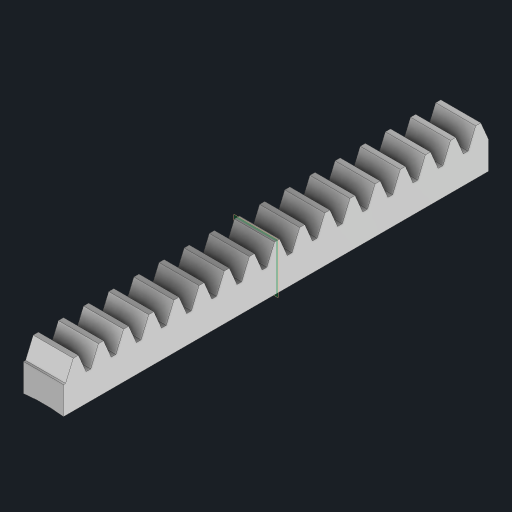
# Autodesk Inventor part: TAPA PRICIPAL CON CREMALLERA
Saved by Autodesk Inventor 2024.3 (Build 283343000, 343)
## iProperties
Created: 2024-06-13
Part Number: TAPA PRICIPAL CON CREMALLERA
Material: Generic
Document SubType Name: Modeling
Designer: Jhuliams
Density: 1 g/cm^3
Appearance: Default
Author: Jhuliams
Autodesk Inventor part; units mm, degrees
ref_plane "YZ Plane" through (0, 0, 0) normal (1, 0, 0) x (0, 1, 0)
ref_plane "XZ Plane" through (0, 0, 0) normal (0, 1, 0) x (-1, 0, 0)
ref_plane "XY Plane" through (0, 0, 0) normal (0, 0, 1) x (1, 0, 0)
sketch "Sketch4" plane through (0, 0, 0) normal (1, 0, 0) x (0, 1, 0)
  line L0 (0, -16.645) -> (0, -21.1217)
  line L1 (3, -17.923) -> (3, -19.8438)
  line L2 (3, -19.8438) -> (-3.75, -22.7192)
  line L3 (0, -21.1217) -> (0, -16.645)
  line L4 (0, -18.8834) -> (0.5045, -18.8834)
  line L5 (3, -17.923) -> (-3.75, -15.0476)
  line L6 (-3.75, 277.1181) -> (-10.75, 277.1181)
  line L7 (-10.75, 277.1181) -> (-10.75, -22.7192)
  line L8 (-10.75, -22.7192) -> (-3.75, -22.7192)
  line L9 (-3.75, -22.7192) -> (-3.75, 277.1181)
  line L10 (0, -7.2203) -> (0, -11.697)
  line L11 (3, -8.4983) -> (3, -10.419)
  line L12 (3, -10.419) -> (-3.75, -13.2945)
  line L13 (0, -11.697) -> (0, -7.2203)
  line L14 (0, -9.4587) -> (0.5045, -9.4587)
  line L15 (3, -8.4983) -> (-3.75, -5.6229)
  line L16 (0, 2.2044) -> (0, -2.2723)
  line L17 (3, 0.9264) -> (3, -0.9943)
  line L18 (3, -0.9943) -> (-3.75, -3.8698)
  line L19 (0, -2.2723) -> (0, 2.2044)
  line L20 (0, -0.034) -> (0.5045, -0.034)
  line L21 (3, 0.9264) -> (-3.75, 3.8018)
  line L22 (0, 11.6291) -> (0, 7.1524)
  line L23 (3, 10.3511) -> (3, 8.4304)
  line L24 (3, 8.4304) -> (-3.75, 5.5549)
  line L25 (0, 7.1524) -> (0, 11.6291)
  line L26 (0, 9.3907) -> (0.5045, 9.3907)
  line L27 (3, 10.3511) -> (-3.75, 13.2265)
  line L28 (0, 21.0538) -> (0, 16.5771)
  line L29 (3, 19.7758) -> (3, 17.8551)
  line L30 (3, 17.8551) -> (-3.75, 14.9796)
  line L31 (0, 16.5771) -> (0, 21.0538)
  line L32 (0, 18.8154) -> (0.5045, 18.8154)
  line L33 (3, 19.7758) -> (-3.75, 22.6512)
  line L34 (0, 30.4785) -> (0, 26.0018)
  line L35 (3, 29.2005) -> (3, 27.2797)
  line L36 (3, 27.2797) -> (-3.75, 24.4043)
  line L37 (0, 26.0018) -> (0, 30.4785)
  line L38 (0, 28.2401) -> (0.5045, 28.2401)
  line L39 (3, 29.2005) -> (-3.75, 32.0759)
  line L40 (0, 39.9032) -> (0, 35.4265)
  line L41 (3, 38.6252) -> (3, 36.7045)
  line L42 (3, 36.7045) -> (-3.75, 33.829)
  line L43 (0, 35.4265) -> (0, 39.9032)
  line L44 (0, 37.6648) -> (0.5045, 37.6648)
  line L45 (3, 38.6252) -> (-3.75, 41.5006)
  line L46 (0, 49.3279) -> (0, 44.8512)
  line L47 (3, 48.0499) -> (3, 46.1292)
  line L48 (3, 46.1292) -> (-3.75, 43.2537)
  line L49 (0, 44.8512) -> (0, 49.3279)
  line L50 (0, 47.0895) -> (0.5045, 47.0895)
  line L51 (3, 48.0499) -> (-3.75, 50.9253)
  line L52 (0, 58.7526) -> (0, 54.2759)
  line L53 (3, 57.4746) -> (3, 55.5539)
  line L54 (3, 55.5539) -> (-3.75, 52.6784)
  line L55 (0, 54.2759) -> (0, 58.7526)
  line L56 (0, 56.5142) -> (0.5045, 56.5142)
  line L57 (3, 57.4746) -> (-3.75, 60.35)
  line L58 (0, 68.1773) -> (0, 63.7006)
  line L59 (3, 66.8993) -> (3, 64.9785)
  line L60 (3, 64.9785) -> (-3.75, 62.1031)
  line L61 (0, 63.7006) -> (0, 68.1773)
  line L62 (0, 65.9389) -> (0.5045, 65.9389)
  line L63 (3, 66.8993) -> (-3.75, 69.7747)
  line L64 (0, 77.602) -> (0, 73.1253)
  line L65 (3, 76.324) -> (3, 74.4032)
  line L66 (3, 74.4032) -> (-3.75, 71.5278)
  line L67 (0, 73.1253) -> (0, 77.602)
  line L68 (0, 75.3636) -> (0.5045, 75.3636)
  line L69 (3, 76.324) -> (-3.75, 79.1994)
  line L70 (0, 87.0267) -> (0, 82.55)
  line L71 (3, 85.7487) -> (3, 83.828)
  line L72 (3, 83.828) -> (-3.75, 80.9525)
  line L73 (0, 82.55) -> (0, 87.0267)
  line L74 (0, 84.7883) -> (0.5045, 84.7883)
  line L75 (3, 85.7487) -> (-3.75, 88.6241)
  line L76 (0, 96.4514) -> (0, 91.9747)
  line L77 (3, 95.1734) -> (3, 93.2527)
  line L78 (3, 93.2527) -> (-3.75, 90.3772)
  line L79 (0, 91.9747) -> (0, 96.4514)
  line L80 (0, 94.213) -> (0.5045, 94.213)
  line L81 (3, 95.1734) -> (-3.75, 98.0488)
  line L82 (0, 105.8761) -> (0, 101.3994)
  line L83 (3, 104.5981) -> (3, 102.6774)
  line L84 (3, 102.6774) -> (-3.75, 99.8019)
  line L85 (0, 101.3994) -> (0, 105.8761)
  line L86 (0, 103.6377) -> (0.5045, 103.6377)
  line L87 (3, 104.5981) -> (-3.75, 107.4735)
  line L88 (0, 115.3008) -> (0, 110.8241)
  line L89 (3, 114.0228) -> (3, 112.1021)
  line L90 (3, 112.1021) -> (-3.75, 109.2266)
  line L91 (0, 110.8241) -> (0, 115.3008)
  line L92 (0, 113.0624) -> (0.5045, 113.0624)
  line L93 (3, 114.0228) -> (-3.75, 116.8982)
  line L94 (0, 124.7255) -> (0, 120.2488)
  line L95 (3, 123.4475) -> (3, 121.5268)
  line L96 (3, 121.5268) -> (-3.75, 118.6513)
  line L97 (0, 120.2488) -> (0, 124.7255)
  line L98 (0, 122.4871) -> (0.5045, 122.4871)
  line L99 (3, 123.4475) -> (-3.75, 126.3229)
  line L100 (0, 134.1502) -> (0, 129.6735)
  line L101 (3, 132.8722) -> (3, 130.9514)
  line L102 (3, 130.9514) -> (-3.75, 128.076)
  line L103 (0, 129.6735) -> (0, 134.1502)
  line L104 (0, 131.9118) -> (0.5045, 131.9118)
  line L105 (3, 132.8722) -> (-3.75, 135.7476)
  line L106 (0, 143.5749) -> (0, 139.0982)
  line L107 (3, 142.2969) -> (3, 140.3761)
  line L108 (3, 140.3761) -> (-3.75, 137.5007)
  line L109 (0, 139.0982) -> (0, 143.5749)
  line L110 (0, 141.3365) -> (0.5045, 141.3365)
  line L111 (3, 142.2969) -> (-3.75, 145.1723)
  line L112 (0, 152.9996) -> (0, 148.5229)
  line L113 (3, 151.7216) -> (3, 149.8008)
  line L114 (3, 149.8008) -> (-3.75, 146.9254)
  line L115 (0, 148.5229) -> (0, 152.9996)
  line L116 (0, 150.7612) -> (0.5045, 150.7612)
  line L117 (3, 151.7216) -> (-3.75, 154.597)
  line L118 (0, 162.4243) -> (0, 157.9476)
  line L119 (3, 161.1463) -> (3, 159.2255)
  line L120 (3, 159.2255) -> (-3.75, 156.3501)
  line L121 (0, 157.9476) -> (0, 162.4243)
  line L122 (0, 160.1859) -> (0.5045, 160.1859)
  line L123 (3, 161.1463) -> (-3.75, 164.0217)
  line L124 (0, 171.849) -> (0, 167.3723)
  line L125 (3, 170.571) -> (3, 168.6502)
  line L126 (3, 168.6502) -> (-3.75, 165.7748)
  line L127 (0, 167.3723) -> (0, 171.849)
  line L128 (0, 169.6106) -> (0.5045, 169.6106)
  line L129 (3, 170.571) -> (-3.75, 173.4464)
  line L130 (0, 181.2737) -> (0, 176.797)
  line L131 (3, 179.9957) -> (3, 178.075)
  line L132 (3, 178.075) -> (-3.75, 175.1995)
  line L133 (0, 176.797) -> (0, 181.2737)
  line L134 (0, 179.0353) -> (0.5045, 179.0353)
  line L135 (3, 179.9957) -> (-3.75, 182.8711)
  line L136 (0, 190.6984) -> (0, 186.2217)
  line L137 (3, 189.4204) -> (3, 187.4997)
  line L138 (3, 187.4997) -> (-3.75, 184.6242)
  line L139 (0, 186.2217) -> (0, 190.6984)
  line L140 (0, 188.46) -> (0.5045, 188.46)
  line L141 (3, 189.4204) -> (-3.75, 192.2958)
  line L142 (0, 200.1231) -> (0, 195.6464)
  line L143 (3, 198.8451) -> (3, 196.9244)
  line L144 (3, 196.9244) -> (-3.75, 194.0489)
  line L145 (0, 195.6464) -> (0, 200.1231)
  line L146 (0, 197.8847) -> (0.5045, 197.8847)
  line L147 (3, 198.8451) -> (-3.75, 201.7205)
  line L148 (0, 209.5478) -> (0, 205.0711)
  line L149 (3, 208.2698) -> (3, 206.3491)
  line L150 (3, 206.3491) -> (-3.75, 203.4736)
  line L151 (0, 205.0711) -> (0, 209.5478)
  line L152 (0, 207.3094) -> (0.5045, 207.3094)
  line L153 (3, 208.2698) -> (-3.75, 211.1452)
  line L154 (0, 218.9725) -> (0, 214.4958)
  line L155 (3, 217.6945) -> (3, 215.7738)
  line L156 (3, 215.7738) -> (-3.75, 212.8983)
  line L157 (0, 214.4958) -> (0, 218.9725)
  line L158 (0, 216.7341) -> (0.5045, 216.7341)
  line L159 (3, 217.6945) -> (-3.75, 220.5699)
  line L160 (0, 228.3972) -> (0, 223.9205)
  line L161 (3, 227.1192) -> (3, 225.1985)
  line L162 (3, 225.1985) -> (-3.75, 222.323)
  line L163 (0, 223.9205) -> (0, 228.3972)
  line L164 (0, 226.1588) -> (0.5045, 226.1588)
  line L165 (3, 227.1192) -> (-3.75, 229.9946)
  line L166 (0, 237.8219) -> (0, 233.3452)
  line L167 (3, 236.5439) -> (3, 234.6232)
  line L168 (3, 234.6232) -> (-3.75, 231.7477)
  line L169 (0, 233.3452) -> (0, 237.8219)
  line L170 (0, 235.5835) -> (0.5045, 235.5835)
  line L171 (3, 236.5439) -> (-3.75, 239.4193)
  line L172 (0, 247.2466) -> (0, 242.7699)
  line L173 (3, 245.9686) -> (3, 244.0479)
  line L174 (3, 244.0479) -> (-3.75, 241.1724)
  line L175 (0, 242.7699) -> (0, 247.2466)
  line L176 (0, 245.0082) -> (0.5045, 245.0082)
  line L177 (3, 245.9686) -> (-3.75, 248.844)
  line L178 (0, 256.6713) -> (0, 252.1946)
  line L179 (3, 255.3933) -> (3, 253.4726)
  line L180 (3, 253.4726) -> (-3.75, 250.5971)
  line L181 (0, 252.1946) -> (0, 256.6713)
  line L182 (0, 254.4329) -> (0.5045, 254.4329)
  line L183 (3, 255.3933) -> (-3.75, 258.2687)
  line L184 (0, 266.096) -> (0, 261.6193)
  line L185 (3, 264.818) -> (3, 262.8972)
  line L186 (3, 262.8972) -> (-3.75, 260.0218)
  line L187 (0, 261.6193) -> (0, 266.096)
  line L188 (0, 263.8576) -> (0.5045, 263.8576)
  line L189 (3, 264.818) -> (-3.75, 267.6934)
  line L190 (0, 275.5207) -> (0, 271.044)
  line L191 (3, 274.2427) -> (3, 272.322)
  line L192 (3, 272.322) -> (-3.75, 269.4465)
  line L193 (0, 271.044) -> (0, 275.5207)
  line L194 (0, 273.2823) -> (0.5045, 273.2823)
  line L195 (3, 274.2427) -> (-3.75, 277.1181)
  line L196 (0, 284.9454) -> (0, 280.4687)
  line L197 (3, 283.6674) -> (3, 281.7466)
  line L198 (3, 281.7466) -> (-3.75, 278.8712)
  line L199 (0, 280.4687) -> (0, 284.9454)
  line L200 (0, 282.707) -> (0.5045, 282.707)
  line L201 (3, 283.6674) -> (-3.75, 286.5428)
  line L202 (0, 294.3701) -> (0, 289.8934)
  line L203 (3, 293.0921) -> (3, 291.1714)
  line L204 (3, 291.1714) -> (-3.75, 288.2959)
  line L205 (0, 289.8934) -> (0, 294.3701)
  line L206 (0, 292.1317) -> (0.5045, 292.1317)
  line L207 (3, 293.0921) -> (-3.75, 295.9675)
  line L208 (0, 303.7948) -> (0, 299.3181)
  line L209 (3, 302.5168) -> (3, 300.596)
  line L210 (3, 300.596) -> (-3.75, 297.7206)
  line L211 (0, 299.3181) -> (0, 303.7948)
  line L212 (0, 301.5564) -> (0.5045, 301.5564)
  line L213 (3, 302.5168) -> (-3.75, 305.3922)
  line L214 (-3.75, 277.1181) -> (-10.75, 277.1181)
  line L215 (-10.75, 277.1181) -> (-10.75, 305.3922)
  line L216 (-10.75, 305.3922) -> (-3.75, 305.3922)
  line L217 (-3.75, 305.3922) -> (-3.75, 277.1181)
  point P0 (-3.75, -22.7192)
  point P1 (-3.75, -13.2945)
  point P2 (-3.75, -3.8698)
  point P3 (-3.75, 5.5549)
  point P4 (-3.75, 14.9796)
  point P5 (-3.75, 24.4043)
  point P6 (-3.75, 33.829)
  point P7 (-3.75, 43.2537)
  point P8 (-3.75, 52.6784)
  point P9 (-3.75, 62.1031)
  point P10 (-3.75, 71.5278)
  point P11 (-3.75, 80.9525)
  point P12 (-3.75, 90.3772)
  point P13 (-3.75, 99.8019)
  point P14 (-3.75, 109.2266)
  point P15 (-3.75, 118.6513)
  point P16 (-3.75, 128.076)
  point P17 (-3.75, 137.5007)
  point P18 (-3.75, 146.9254)
  point P19 (-3.75, 156.3501)
  point P20 (-3.75, 165.7748)
  point P21 (-3.75, 175.1995)
  point P22 (-3.75, 184.6242)
  point P23 (-3.75, 194.0489)
  point P24 (-3.75, 203.4736)
  point P25 (-3.75, 212.8983)
  point P26 (-3.75, 222.323)
  point P27 (-3.75, 231.7477)
  point P28 (-3.75, 241.1724)
  point P29 (-3.75, 250.5971)
  point P30 (-3.75, 260.0218)
  point P31 (-3.75, 269.4465)
  point P32 (-3.75, 278.8712)
  point P33 (-3.75, 288.2959)
  point P34 (-3.75, 297.7206)
  point P35 (-3.75, 156.3501)
  point P36 (-3.75, 165.7748)
  point P37 (-3.75, 175.1995)
  point P38 (-3.75, 184.6242)
  point P39 (-3.75, 194.0489)
  point P40 (-3.75, 203.4736)
  point P41 (-3.75, 212.8983)
  point P42 (-3.75, 222.323)
  point P43 (-3.75, 231.7477)
  point P44 (-3.75, 241.1724)
  point P45 (-3.75, 250.5971)
  point P46 (-3.75, 260.0218)
  point P47 (-3.75, 269.4465)
  point P48 (-3.75, 278.8712)
  point P49 (-3.75, 288.2959)
  point P50 (-3.75, 297.7206)
  point P51 (-3.75, -13.2945)
  point P52 (-3.75, -3.8698)
  point P53 (-3.75, 5.5549)
  point P54 (-3.75, 14.9796)
  point P55 (-3.75, 24.4043)
  point P56 (-3.75, 33.829)
  point P57 (-3.75, 43.2537)
  point P58 (-3.75, 52.6784)
  point P59 (-3.75, 62.1031)
  point P60 (-3.75, 71.5278)
  point P61 (-3.75, 80.9525)
  point P62 (-3.75, 90.3772)
  point P63 (-3.75, 99.8019)
  point P64 (-3.75, 109.2266)
  point P65 (-3.75, 118.6513)
  point P66 (-3.75, 128.076)
  point P67 (-3.75, 137.5007)
  point P68 (-3.75, 146.9254)
  dimension "d53" = 3
  dimension "d56" = 4.4767
  dimension "d66" = 7
  dimension "d76" = 9.4247
  dimension "d81" = 7
  constraints: 434 end point, 70 point on line, 4 parallel, 3 horizontal, 3 vertical, 2 perpendicular, 1 collinear, 1 midpoint, 1 symmetric about line, 512 other
  measures "d53" distance between parallel lines of L0 L1
  measures "d56" distance of L0.start L0.end
  measures "d66" distance of L8.end L7.end
  measures "d76" distance of L0.start L10.start
  measures "d81" distance of L215.end L216.end
extrude "Extrusion2" add sketch "Sketch4" along normal mid plane 15
sketch "Sketch7" plane through (-7.5, -10.75, -22.7192) normal (0, -1, 0) x (1, 0, 0)
  line L0 (0, 0) -> (15, 0) projected
  line L1 (82.5, 250) -> (-67.5, 250)
  line L2 (-67.5, 250) -> (-67.5, -250)
  line L3 (-67.5, -250) -> (82.5, -250)
  line L4 (82.5, -250) -> (82.5, 250)
  line L5 (82.5, 250) -> (-67.5, -250) construction
  line L6 (-67.5, 250) -> (82.5, -250) construction
  line L7 (82.5, 0) -> (-67.5, 0)
  point P0 (7.5, 0)
  point P1 (15, 0)
  dimension "d82" = 150
  dimension "d83" = 500
  constraints: 14 end point, 5 midpoint, 2 parallel, 1 horizontal, 1 perpendicular
  measures "d82" distance of L3.end L2.end
  measures "d83" distance of L2.end L1.end
extrude "Extrusion5" add sketch "Sketch7" along normal blind 5 contours L7 L2 L1 L4 L0
sketch "Sketch8" plane through (-7.5, -10.75, 305.3922) normal (0, 0, 1) x (1, 0, 0)
  line L0 (82.5, -5) -> (-67.5, -5) projected
  line L1 (15, 0) -> (0, 0)
  line L2 (0, 0) -> (0, -5)
  line L3 (0, -5) -> (15, -5)
  line L4 (15, -5) -> (15, 0)
  point P0 (7.5, 10.75)
  constraints: 8 end point, 2 parallel, 1 horizontal, 1 perpendicular, 1 point on line
extrude "Extrusion6" add sketch "Sketch8" against normal blind 90
fillet "Fillet3" radius 10 2 edges at (-7.5, -10.75, 102.2808) (7.5, -10.75, 102.2808)
sketch "Sketch9" plane through (75, -15.75, -22.7192) normal (0, 0, -1) x (-1, 0, 0)
  line L0 (82.9606, 12) -> (67.0394, 12) projected
  arc A0 (57.5, 5) -> (67.0394, 12) centre (57.5, 15) ccw projected
  line L1 (57.5, 5) -> (0, 5) projected
  line L2 (0, 5) -> (0, 0) projected
  line L3 (150, 0) -> (0, 0) projected
  line L4 (150, 5) -> (150, 0) projected
  line L5 (150, 5) -> (92.5, 5) projected
  arc A1 (82.9606, 12) -> (92.5, 5) centre (92.5, 15) ccw projected
  line L6 (82.5, 18.75) -> (82.5, 15) projected
  line L7 (82.5, 18.75) -> (67.5, 18.75) projected
  line L8 (67.5, 15) -> (67.5, 18.75) projected
  arc A2 (67.0394, 12) -> (67.5, 15) centre (57.5, 15) ccw projected
  line L9 (82.9606, 12) -> (67.0394, 12) projected
  arc A3 (82.5, 15) -> (82.9606, 12) centre (92.5, 15) ccw projected
  line L10 (82.5, 18.75) -> (67.5, 18.75)
  line L11 (67.5, 18.75) -> (67.5, 1.6)
  line L12 (67.5, 1.6) -> (82.5, 1.6)
  line L13 (82.5, 1.6) -> (82.5, 18.75)
  point P0 (75, 15.75)
  dimension "d87" = 1.6
  constraints: 8 end point, 2 parallel, 1 horizontal, 1 perpendicular
  measures "d87" distance between parallel lines of L3 L12
extrude "Extrusion7" cut sketch "Sketch9" against normal up to surface (250 mm away) contours A1 L5 L4 L3 L2 L1 A0 L0 L11 L12 L13 | L0 L13 A3 | L0 A2 L11
sketch "Sketch11" plane through (-7.5, -3.75, 305.3922) normal (0, 0, 1) x (1, 0, 0)
  line L0 (15, 0) -> (15, -12) projected
  line L1 (0, 0) -> (15, 0) projected
  line L2 (0, 0) -> (0, -12) projected
  line L3 (0, -12) -> (15, -12) projected
  line L4 (0, -10.4) -> (15, -10.4) projected
  line L5 (15, -10.4) -> (0, -10.4) projected
  arc A0 (15, -10.4) -> (0, -10.4) centre (7.5, -69.4254) ccw
  point P0 (7.5, 3.75)
  dimension "d93" = 59.5
  constraints: 2 point on circle, 1 centre point
  measures "d93" radius of A0
extrude "Extrusion9" cut sketch "Sketch11" against normal through all contours L0 L3 L2 L4 | L4 A0
sketch "Sketch12" plane through (7.5, 0, 0) normal (1, 0, 0) x (0, 0, -1)
  line L0 (-305.3922, -14.15) -> (22.7192, -14.15) projected
  line L1 (22.7192, -3.75) -> (22.7192, -14.15) projected
  line L2 (22.7192, -3.75) -> (19.8438, 3) projected
  line L3 (19.8438, 3) -> (17.923, 3) projected
  line L4 (17.923, 3) -> (15.0476, -3.75) projected
  line L5 (13.2945, -3.75) -> (15.0476, -3.75) projected
  line L6 (13.2945, -3.75) -> (10.419, 3) projected
  line L7 (10.419, 3) -> (8.4983, 3) projected
  line L8 (8.4983, 3) -> (5.6229, -3.75) projected
  line L9 (3.8698, -3.75) -> (5.6229, -3.75) projected
  line L10 (3.8698, -3.75) -> (0.9943, 3) projected
  line L11 (0.9943, 3) -> (-0.9264, 3) projected
  line L12 (-0.9264, 3) -> (-3.8018, -3.75) projected
  line L13 (-5.5549, -3.75) -> (-3.8018, -3.75) projected
  line L14 (-5.5549, -3.75) -> (-8.4304, 3) projected
  line L15 (-8.4304, 3) -> (-10.3511, 3) projected
  line L16 (-10.3511, 3) -> (-13.2265, -3.75) projected
  line L17 (-14.9796, -3.75) -> (-13.2265, -3.75) projected
  line L18 (-14.9796, -3.75) -> (-17.8551, 3) projected
  line L19 (-17.8551, 3) -> (-19.7758, 3) projected
  line L20 (-19.7758, 3) -> (-22.6512, -3.75) projected
  line L21 (-24.4043, -3.75) -> (-22.6512, -3.75) projected
  line L22 (-24.4043, -3.75) -> (-27.2798, 3) projected
  line L23 (-27.2798, 3) -> (-29.2005, 3) projected
  line L24 (-29.2005, 3) -> (-32.0759, -3.75) projected
  line L25 (-33.829, -3.75) -> (-32.0759, -3.75) projected
  line L26 (-33.829, -3.75) -> (-36.7045, 3) projected
  line L27 (-36.7045, 3) -> (-38.6252, 3) projected
  line L28 (-38.6252, 3) -> (-41.5006, -3.75) projected
  line L29 (-43.2537, -3.75) -> (-41.5006, -3.75) projected
  line L30 (-43.2537, -3.75) -> (-46.1292, 3) projected
  line L31 (-46.1292, 3) -> (-48.0499, 3) projected
  line L32 (-48.0499, 3) -> (-50.9253, -3.75) projected
  line L33 (-52.6784, -3.75) -> (-50.9253, -3.75) projected
  line L34 (-52.6784, -3.75) -> (-55.5539, 3) projected
  line L35 (-55.5539, 3) -> (-57.4746, 3) projected
  line L36 (-57.4746, 3) -> (-60.35, -3.75) projected
  line L37 (-62.1031, -3.75) -> (-60.35, -3.75) projected
  line L38 (-62.1031, -3.75) -> (-64.9785, 3) projected
  line L39 (-64.9785, 3) -> (-66.8993, 3) projected
  line L40 (-66.8993, 3) -> (-69.7747, -3.75) projected
  line L41 (-71.5278, -3.75) -> (-69.7747, -3.75) projected
  line L42 (-71.5278, -3.75) -> (-74.4032, 3) projected
  line L43 (-74.4032, 3) -> (-76.324, 3) projected
  line L44 (-76.324, 3) -> (-79.1994, -3.75) projected
  line L45 (-80.9525, -3.75) -> (-79.1994, -3.75) projected
  line L46 (-80.9525, -3.75) -> (-83.828, 3) projected
  line L47 (-83.828, 3) -> (-85.7487, 3) projected
  line L48 (-85.7487, 3) -> (-88.6241, -3.75) projected
  line L49 (-90.3772, -3.75) -> (-88.6241, -3.75) projected
  line L50 (-90.3772, -3.75) -> (-93.2527, 3) projected
  line L51 (-93.2527, 3) -> (-95.1734, 3) projected
  line L52 (-95.1734, 3) -> (-98.0488, -3.75) projected
  line L53 (-99.8019, -3.75) -> (-98.0488, -3.75) projected
  line L54 (-99.8019, -3.75) -> (-102.6774, 3) projected
  line L55 (-102.6774, 3) -> (-104.5981, 3) projected
  line L56 (-104.5981, 3) -> (-107.4735, -3.75) projected
  line L57 (-109.2266, -3.75) -> (-107.4735, -3.75) projected
  line L58 (-109.2266, -3.75) -> (-112.1021, 3) projected
  line L59 (-112.1021, 3) -> (-114.0228, 3) projected
  line L60 (-114.0228, 3) -> (-116.8982, -3.75) projected
  line L61 (-118.6513, -3.75) -> (-116.8982, -3.75) projected
  line L62 (-118.6513, -3.75) -> (-121.5268, 3) projected
  line L63 (-121.5268, 3) -> (-123.4475, 3) projected
  line L64 (-123.4475, 3) -> (-126.3229, -3.75) projected
  line L65 (-128.076, -3.75) -> (-126.3229, -3.75) projected
  line L66 (-128.076, -3.75) -> (-130.9514, 3) projected
  line L67 (-130.9514, 3) -> (-132.8722, 3) projected
  line L68 (-132.8722, 3) -> (-135.7476, -3.75) projected
  line L69 (-137.5007, -3.75) -> (-135.7476, -3.75) projected
  line L70 (-137.5007, -3.75) -> (-140.3761, 3) projected
  line L71 (-140.3761, 3) -> (-142.2969, 3) projected
  line L72 (-142.2969, 3) -> (-145.1723, -3.75) projected
  line L73 (-146.9254, -3.75) -> (-145.1723, -3.75) projected
  line L74 (-146.9254, -3.75) -> (-149.8008, 3) projected
  line L75 (-149.8008, 3) -> (-151.7216, 3) projected
  line L76 (-151.7216, 3) -> (-154.597, -3.75) projected
  line L77 (-156.3501, -3.75) -> (-154.597, -3.75) projected
  line L78 (-156.3501, -3.75) -> (-159.2255, 3) projected
  line L79 (-159.2255, 3) -> (-161.1463, 3) projected
  line L80 (-161.1463, 3) -> (-164.0217, -3.75) projected
  line L81 (-165.7748, -3.75) -> (-164.0217, -3.75) projected
  line L82 (-165.7748, -3.75) -> (-168.6502, 3) projected
  line L83 (-168.6502, 3) -> (-170.571, 3) projected
  line L84 (-170.571, 3) -> (-173.4464, -3.75) projected
  line L85 (-175.1995, -3.75) -> (-173.4464, -3.75) projected
  line L86 (-175.1995, -3.75) -> (-178.075, 3) projected
  line L87 (-178.075, 3) -> (-179.9957, 3) projected
  line L88 (-179.9957, 3) -> (-182.8711, -3.75) projected
  line L89 (-184.6242, -3.75) -> (-182.8711, -3.75) projected
  line L90 (-184.6242, -3.75) -> (-187.4997, 3) projected
  line L91 (-187.4997, 3) -> (-189.4204, 3) projected
  line L92 (-189.4204, 3) -> (-192.2958, -3.75) projected
  line L93 (-194.0489, -3.75) -> (-192.2958, -3.75) projected
  line L94 (-194.0489, -3.75) -> (-196.9244, 3) projected
  line L95 (-196.9244, 3) -> (-198.8451, 3) projected
  line L96 (-198.8451, 3) -> (-201.7205, -3.75) projected
  line L97 (-203.4736, -3.75) -> (-201.7205, -3.75) projected
  line L98 (-203.4736, -3.75) -> (-206.3491, 3) projected
  line L99 (-206.3491, 3) -> (-208.2698, 3) projected
  line L100 (-208.2698, 3) -> (-211.1452, -3.75) projected
  line L101 (-212.8983, -3.75) -> (-211.1452, -3.75) projected
  line L102 (-212.8983, -3.75) -> (-215.7738, 3) projected
  line L103 (-215.7738, 3) -> (-217.6945, 3) projected
  line L104 (-217.6945, 3) -> (-220.5699, -3.75) projected
  line L105 (-222.323, -3.75) -> (-220.5699, -3.75) projected
  line L106 (-222.323, -3.75) -> (-225.1985, 3) projected
  line L107 (-225.1985, 3) -> (-227.1192, 3) projected
  line L108 (-227.1192, 3) -> (-229.9946, -3.75) projected
  line L109 (-229.9946, -3.75) -> (-231.7477, -3.75) projected
  line L110 (-231.7477, -3.75) -> (-234.6232, 3) projected
  line L111 (-234.6232, 3) -> (-236.5439, 3) projected
  line L112 (-236.5439, 3) -> (-239.4193, -3.75) projected
  line L113 (-239.4193, -3.75) -> (-241.1724, -3.75) projected
  line L114 (-241.1724, -3.75) -> (-244.0479, 3) projected
  line L115 (-244.0479, 3) -> (-245.9686, 3) projected
  line L116 (-245.9686, 3) -> (-248.844, -3.75) projected
  line L117 (-248.844, -3.75) -> (-250.5971, -3.75) projected
  line L118 (-250.5971, -3.75) -> (-253.4726, 3) projected
  line L119 (-253.4726, 3) -> (-255.3933, 3) projected
  line L120 (-255.3933, 3) -> (-258.2687, -3.75) projected
  line L121 (-258.2687, -3.75) -> (-260.0218, -3.75) projected
  line L122 (-260.0218, -3.75) -> (-262.8972, 3) projected
  line L123 (-262.8972, 3) -> (-264.818, 3) projected
  line L124 (-264.818, 3) -> (-267.6934, -3.75) projected
  line L125 (-267.6934, -3.75) -> (-269.4465, -3.75) projected
  line L126 (-269.4465, -3.75) -> (-272.322, 3) projected
  line L127 (-272.322, 3) -> (-274.2427, 3) projected
  line L128 (-274.2427, 3) -> (-277.1181, -3.75) projected
  line L129 (-277.1181, -3.75) -> (-278.8712, -3.75) projected
  line L130 (-278.8712, -3.75) -> (-281.7466, 3) projected
  line L131 (-281.7466, 3) -> (-283.6674, 3) projected
  line L132 (-283.6674, 3) -> (-286.5428, -3.75) projected
  line L133 (-286.5428, -3.75) -> (-288.2959, -3.75) projected
  line L134 (-288.2959, -3.75) -> (-291.1714, 3) projected
  line L135 (-291.1714, 3) -> (-293.0921, 3) projected
  line L136 (-293.0921, 3) -> (-295.9675, -3.75) projected
  line L137 (-295.9675, -3.75) -> (-297.7206, -3.75) projected
  line L138 (-297.7206, -3.75) -> (-300.596, 3) projected
  line L139 (-300.596, 3) -> (-302.5168, 3) projected
  line L140 (-302.5168, 3) -> (-305.3922, -3.75) projected
  line L141 (-305.3922, -3.75) -> (-305.3922, -14.15) projected
  line L142 (-305.3922, -14.15) -> (-136.5124, -14.15)
  line L143 (-136.5124, -14.15) -> (-136.5124, 36.402)
  line L144 (-136.5124, 36.402) -> (-305.3922, 36.402)
  line L145 (-305.3922, 36.402) -> (-305.3922, -14.15)
  line L146 (-136.5124, 36.402) -> (22.7192, 36.402)
  line L147 (22.7192, 36.402) -> (22.7192, -14.15)
  line L148 (22.7192, -14.15) -> (-136.5124, -14.15)
  line L149 (-136.5124, -14.15) -> (-136.5124, 36.402)
  point P0 (0, 0)
  point P1 (-136.5124, -14.15)
  constraints: 16 end point, 4 parallel, 2 horizontal, 2 perpendicular
extrude "Extrusion10" cut sketch "Sketch12" against normal through all contours L141 L140 L139 L138 L137 L136 L135 L134 L133 L132 L131 L130 L129 L128 L127 L126 L125 L124 L123 L122 L121 L120 L119 L118 L117 L116 L115 L114 L113 L112 L111 L110 L109 L108 L107 L106 L105 L104 L103 L102 L101 L100 L99 L98 L97 L96 L95 L94 L93 L92 L91 L90 L89 L88 L87 L86 L85 L84 L83 L82 L81 L80 L79 L78 L77 L76 L75 L74 L73 L72 L71 L70 L69 L143 L0 | L145 L144 L143 L69 L70 L71 L72 L73 L74 L75 L76 L77 L78 L79 L80 L81 L82 L83 L84 L85 L86 L87 L88 L89 L90 L91 L92 L93 L94 L95 L96 L97 L98 L99 L100 L101 L102 L103 L104 L105 L106 L107 L108 L109 L110 L111 L112 L113 L114 L115 L116 L117 L118 L119 L120 L121 L122 L123 L124 L125 L126 L127 L128 L129 L130 L131 L132 L133 L134 L135 L136 L137 L138 L139 L140
ref_plane "Work Plane1" through (7.5, -3.75, 56.8966) normal (0, 0, -1) x (-1, 0, 0)
sketch "Sketch10" plane through (-7.5, 0, 0) normal (-1, 0, 0) x (0, 0, 1)
  line L0 (107.4735, -3.75) -> (104.5981, 3) projected
  line L1 (104.5981, 3) -> (102.6774, 3) projected
  line L2 (102.6774, 3) -> (99.8019, -3.75) projected
  line L3 (98.0488, -3.75) -> (99.8019, -3.75) projected
  line L4 (98.0488, -3.75) -> (95.1734, 3) projected
  line L5 (95.1734, 3) -> (93.2527, 3) projected
  line L6 (93.2527, 3) -> (90.3772, -3.75) projected
  line L7 (88.6241, -3.75) -> (90.3772, -3.75) projected
  line L8 (88.6241, -3.75) -> (85.7487, 3) projected
  line L9 (85.7487, 3) -> (83.828, 3) projected
  line L10 (83.828, 3) -> (80.9525, -3.75) projected
  line L11 (79.1994, -3.75) -> (80.9525, -3.75) projected
  line L12 (79.1994, -3.75) -> (76.324, 3) projected
  line L13 (76.324, 3) -> (74.4032, 3) projected
  line L14 (74.4032, 3) -> (71.5278, -3.75) projected
  line L15 (69.7747, -3.75) -> (71.5278, -3.75) projected
  line L16 (69.7747, -3.75) -> (66.8993, 3) projected
  line L17 (66.8993, 3) -> (64.9785, 3) projected
  line L18 (64.9785, 3) -> (62.1031, -3.75) projected
  line L19 (60.35, -3.75) -> (62.1031, -3.75) projected
  line L20 (60.35, -3.75) -> (57.4746, 3) projected
  line L21 (57.4746, 3) -> (55.5539, 3) projected
  line L22 (55.5539, 3) -> (52.6784, -3.75) projected
  line L23 (50.9253, -3.75) -> (52.6784, -3.75) projected
  line L24 (50.9253, -3.75) -> (48.0499, 3) projected
  line L25 (48.0499, 3) -> (46.1292, 3) projected
  line L26 (46.1292, 3) -> (43.2537, -3.75) projected
  line L27 (41.5006, -3.75) -> (43.2537, -3.75) projected
  line L28 (41.5006, -3.75) -> (38.6252, 3) projected
  line L29 (38.6252, 3) -> (36.7045, 3) projected
  line L30 (36.7045, 3) -> (33.829, -3.75) projected
  line L31 (32.0759, -3.75) -> (33.829, -3.75) projected
  line L32 (32.0759, -3.75) -> (29.2005, 3) projected
  line L33 (29.2005, 3) -> (27.2798, 3) projected
  line L34 (27.2798, 3) -> (24.4043, -3.75) projected
  line L35 (22.6512, -3.75) -> (24.4043, -3.75) projected
  line L36 (22.6512, -3.75) -> (19.7758, 3) projected
  line L37 (19.7758, 3) -> (17.8551, 3) projected
  line L38 (17.8551, 3) -> (14.9796, -3.75) projected
  line L39 (13.2265, -3.75) -> (14.9796, -3.75) projected
  line L40 (13.2265, -3.75) -> (10.3511, 3) projected
  line L41 (10.3511, 3) -> (8.4304, 3) projected
  line L42 (8.4304, 3) -> (5.5549, -3.75) projected
  line L43 (3.8018, -3.75) -> (5.5549, -3.75) projected
  line L44 (3.8018, -3.75) -> (0.9264, 3) projected
  line L45 (0.9264, 3) -> (-0.9943, 3) projected
  line L46 (-0.9943, 3) -> (-3.8698, -3.75) projected
  line L47 (-5.6229, -3.75) -> (-3.8698, -3.75) projected
  line L48 (-5.6229, -3.75) -> (-8.4983, 3) projected
  line L49 (-8.4983, 3) -> (-10.419, 3) projected
  line L50 (-10.419, 3) -> (-13.2945, -3.75) projected
  line L51 (-15.0476, -3.75) -> (-13.2945, -3.75) projected
  line L52 (-15.0476, -3.75) -> (-17.923, 3) projected
  line L53 (-17.923, 3) -> (-19.8438, 3) projected
  line L54 (-19.8438, 3) -> (-22.7192, -3.75) projected
  line L55 (-22.7192, -14.15) -> (-22.7192, -3.75) projected
  line L56 (-22.7192, -14.15) -> (227.2808, -14.15) projected
  line L57 (227.2808, -15.75) -> (227.2808, -14.15) projected
  line L58 (305.3922, -15.75) -> (227.2808, -15.75) projected
  line L59 (305.3922, -3.75) -> (305.3922, -15.75) projected
  line L60 (305.3922, -3.75) -> (302.5168, 3) projected
  line L61 (302.5168, 3) -> (300.596, 3) projected
  line L62 (300.596, 3) -> (297.7206, -3.75) projected
  line L63 (297.7206, -3.75) -> (295.9675, -3.75) projected
  line L64 (295.9675, -3.75) -> (293.0921, 3) projected
  line L65 (293.0921, 3) -> (291.1714, 3) projected
  line L66 (291.1714, 3) -> (288.2959, -3.75) projected
  line L67 (288.2959, -3.75) -> (286.5428, -3.75) projected
  line L68 (286.5428, -3.75) -> (283.6674, 3) projected
  line L69 (283.6674, 3) -> (281.7466, 3) projected
  line L70 (281.7466, 3) -> (278.8712, -3.75) projected
  line L71 (278.8712, -3.75) -> (277.1181, -3.75) projected
  line L72 (277.1181, -3.75) -> (274.2427, 3) projected
  line L73 (274.2427, 3) -> (272.322, 3) projected
  line L74 (272.322, 3) -> (269.4465, -3.75) projected
  line L75 (269.4465, -3.75) -> (267.6934, -3.75) projected
  line L76 (267.6934, -3.75) -> (264.818, 3) projected
  line L77 (264.818, 3) -> (262.8972, 3) projected
  line L78 (262.8972, 3) -> (260.0218, -3.75) projected
  line L79 (260.0218, -3.75) -> (258.2687, -3.75) projected
  line L80 (258.2687, -3.75) -> (255.3933, 3) projected
  line L81 (255.3933, 3) -> (253.4726, 3) projected
  line L82 (253.4726, 3) -> (250.5971, -3.75) projected
  line L83 (250.5971, -3.75) -> (248.844, -3.75) projected
  line L84 (248.844, -3.75) -> (245.9686, 3) projected
  line L85 (245.9686, 3) -> (244.0479, 3) projected
  line L86 (244.0479, 3) -> (241.1724, -3.75) projected
  line L87 (241.1724, -3.75) -> (239.4193, -3.75) projected
  line L88 (239.4193, -3.75) -> (236.5439, 3) projected
  line L89 (236.5439, 3) -> (234.6232, 3) projected
  line L90 (234.6232, 3) -> (231.7477, -3.75) projected
  line L91 (231.7477, -3.75) -> (229.9946, -3.75) projected
  line L92 (229.9946, -3.75) -> (227.1192, 3) projected
  line L93 (227.1192, 3) -> (225.1985, 3) projected
  line L94 (225.1985, 3) -> (222.323, -3.75) projected
  line L95 (220.5699, -3.75) -> (222.323, -3.75) projected
  line L96 (220.5699, -3.75) -> (217.6945, 3) projected
  line L97 (217.6945, 3) -> (215.7738, 3) projected
  line L98 (215.7738, 3) -> (212.8983, -3.75) projected
  line L99 (211.1452, -3.75) -> (212.8983, -3.75) projected
  line L100 (211.1452, -3.75) -> (208.2698, 3) projected
  line L101 (208.2698, 3) -> (206.3491, 3) projected
  line L102 (206.3491, 3) -> (203.4736, -3.75) projected
  line L103 (201.7205, -3.75) -> (203.4736, -3.75) projected
  line L104 (201.7205, -3.75) -> (198.8451, 3) projected
  line L105 (198.8451, 3) -> (196.9244, 3) projected
  line L106 (196.9244, 3) -> (194.0489, -3.75) projected
  line L107 (192.2958, -3.75) -> (194.0489, -3.75) projected
  line L108 (192.2958, -3.75) -> (189.4204, 3) projected
  line L109 (189.4204, 3) -> (187.4997, 3) projected
  line L110 (187.4997, 3) -> (184.6242, -3.75) projected
  line L111 (182.8711, -3.75) -> (184.6242, -3.75) projected
  line L112 (182.8711, -3.75) -> (179.9957, 3) projected
  line L113 (179.9957, 3) -> (178.075, 3) projected
  line L114 (178.075, 3) -> (175.1995, -3.75) projected
  line L115 (173.4464, -3.75) -> (175.1995, -3.75) projected
  line L116 (173.4464, -3.75) -> (170.571, 3) projected
  line L117 (170.571, 3) -> (168.6502, 3) projected
  line L118 (168.6502, 3) -> (165.7748, -3.75) projected
  line L119 (164.0217, -3.75) -> (165.7748, -3.75) projected
  line L120 (164.0217, -3.75) -> (161.1463, 3) projected
  line L121 (161.1463, 3) -> (159.2255, 3) projected
  line L122 (159.2255, 3) -> (156.3501, -3.75) projected
  line L123 (154.597, -3.75) -> (156.3501, -3.75) projected
  line L124 (154.597, -3.75) -> (151.7216, 3) projected
  line L125 (151.7216, 3) -> (149.8008, 3) projected
  line L126 (149.8008, 3) -> (146.9254, -3.75) projected
  line L127 (145.1723, -3.75) -> (146.9254, -3.75) projected
  line L128 (145.1723, -3.75) -> (142.2969, 3) projected
  line L129 (142.2969, 3) -> (140.3761, 3) projected
  line L130 (140.3761, 3) -> (137.5007, -3.75) projected
  line L131 (135.7476, -3.75) -> (137.5007, -3.75) projected
  line L132 (135.7476, -3.75) -> (132.8722, 3) projected
  line L133 (132.8722, 3) -> (130.9514, 3) projected
  line L134 (130.9514, 3) -> (128.076, -3.75) projected
  line L135 (126.3229, -3.75) -> (128.076, -3.75) projected
  line L136 (126.3229, -3.75) -> (123.4475, 3) projected
  line L137 (123.4475, 3) -> (121.5268, 3) projected
  line L138 (121.5268, 3) -> (118.6513, -3.75) projected
  line L139 (116.8982, -3.75) -> (118.6513, -3.75) projected
  line L140 (116.8982, -3.75) -> (114.0228, 3) projected
  line L141 (114.0228, 3) -> (112.1021, 3) projected
  line L142 (112.1021, 3) -> (109.2266, -3.75) projected
  line L143 (107.4735, -3.75) -> (109.2266, -3.75) projected
  line L144 (-22.7192, -14.15) -> (43.2537, -14.15)
  line L145 (43.2537, -14.15) -> (43.2537, 6.742)
  line L146 (43.2537, 6.742) -> (-22.7192, 6.742)
  line L147 (-22.7192, 6.742) -> (-22.7192, -14.15)
  point P0 (0, 0)
  constraints: 8 end point, 2 parallel, 1 horizontal, 1 perpendicular, 1 point on line
body "Solid2"
